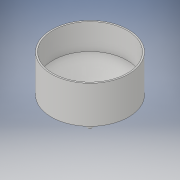
# Autodesk Inventor part: Embudo
Saved by Autodesk Inventor 2019 (Build 230136000, 136)
## iProperties
Created: 2020-02-03
Part Number: Embudo
Material: Generic
Document SubType Name: Modeling
Designer: Sergio
Density: 1 g/cm^3
Appearance: Default
Author: Sergio
Autodesk Inventor part; units mm, degrees
ref_plane "YZ Plane" through (0, 0, 0) normal (1, 0, 0) x (0, 1, 0)
ref_plane "XZ Plane" through (0, 0, 0) normal (0, 1, 0) x (-1, 0, 0)
ref_plane "XY Plane" through (0, 0, 0) normal (0, 0, 1) x (1, 0, 0)
sketch "Sketch1" plane through (0, 0, 0) normal (1, 0, 0) x (0, 1, 0)
  line L0 (0, 0) -> (0, 50) construction
  line L1 (9.4003, 53.5165) -> (0, 53.5165)
  line L2 (0, 45.2) -> (6.2643, 45.2)
  line L3 (0, 48.85) -> (6.8149, 48.85)
  line L4 (6.8149, 48.85) -> (6.8149, 51.15)
  line L5 (6.8149, 51.15) -> (0, 51.15)
  line L6 (-58.3405, 0) -> (70.0432, 0) projected
  line L7 (15.7583, 51.5165) -> (-36.8757, 1.8)
  line L8 (-36.8757, 1.8) -> (-40, 1.5)
  line L9 (6.2643, 45.2) -> (-40, 1.5)
  line L10 (0, 53.5165) -> (0, 51.15)
  line L11 (0, 48.85) -> (0, 45.2)
  line L12 (9.4003, 53.5165) -> (51.7027, 53.5165)
  line L13 (51.7027, 53.5165) -> (51.7027, 51.5165)
  line L14 (51.7027, 51.5165) -> (15.7583, 51.5165)
  point P0 (41.9924, 78.9477)
  dimension "d0" = 50
  dimension "d10" = 1.8
  dimension "d11" = 1.5
  dimension "d13" = 2
  constraints: 28 end point, 5 perpendicular, 3 horizontal, 3 parallel, 2 point on line, 1 vertical
  measures "d0" distance of L0.start L0.end
  measures "d10" distance from line of L6 L7.end
  measures "d11" distance from line of L6 L8.end
  measures "d13" distance of L12.end L13.end
revolve "Revolution1" add sketch "Sketch1" angle 360 about axis through (0, -10, 0) along (0, 1, 0)
body "Solid1"
